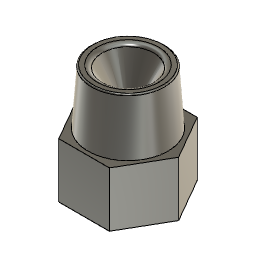
TubeNut175 (Autodesk Fusion 360 design; units mm, degrees)
Autodesk Fusion 360 part; units mm, degrees
note: some values were not read from the file. Set by a fixed rule: which sketch regions a step uses.
sketch "Sketch1" plane through (0, 0, 0) normal (0, 1, 0) x (1, 0, 0)
  circle A0 centre (0, 0) radius 8
  circle A1 centre (0, 0) radius 4
  circle A2 centre (0, 0) radius 1
  line L0 (4.6188, -8) -> (9.2376, 0)
  line L1 (9.2376, 0) -> (4.6188, 8)
  line L2 (4.6188, 8) -> (-4.6188, 8)
  line L3 (-4.6188, 8) -> (-9.2376, 0)
  line L4 (-9.2376, 0) -> (-4.6188, -8)
  line L5 (-4.6188, -8) -> (4.6188, -8)
  dimension "d1_1" = 16
  dimension "d4_1" = 8
  dimension "d7_1" = 2
  constraint coincident A0.centre A1.centre
  constraint concentric A0 A1
  measures "d1_1" diameter of A0
  measures "d4_1" diameter of A1
  measures "d7_1" diameter of A2
extrude "Extrude1" add sketch "Sketch1" along normal blind 20 draft -4 contours A0 | A1 | A2
extrude "Extrude4" add sketch "Sketch1" along normal blind 10 contours A0 | A0 L0 L1 | A0 L1 L2 | A0 L0 L5 | A0 L2 L3 | A0 L4 L5 | A0 L3 L4 | A1 | A2
extrude "Extrude3" cut sketch "Sketch1" along normal through all contours A2
chamfer "Chamfer1" distance 4 angle 60 1 edges at (-0.9323, 20, -0.3616) measured on face at (4.706, 20, -0.3776)
fillet "Fillet1" radius 1 1 edges at (-4.6616, 20, 1.8081)
fillet "Fillet2" radius 3 1 edges at (-0.9323, 13.0718, -0.3616)
fillet "Fillet3" radius 0.25 1 edges at (-6.1547, 20, -2.3872)
sketch "Sketch2" plane through (0, 0, 0) normal (0, 0, 1) x (1, 0, 0)
  line L0 (0, 24) -> (0, -24) construction
  line L1 (-21.801, 0) -> (21.801, 0) construction
  line L2 (-4.5, 0) -> (-4.5, 8)
  line L3 (-4.5, 8) -> (0, 12.5)
  line L4 (0, 12.5) -> (0, 0)
  line L5 (-4.5, 0) -> (0, 0)
  dimension "d16" = 45
  dimension "d17" = 4.5
  dimension "d23" = 8
  constraint horizontal L1
  constraint vertical L0
  constraint coincident L4.end L5.end
  constraint coincident L0 L3.end
  constraint midpoint L4.end L1
  constraint perpendicular L0 L5
  constraint midpoint L4.end L0
  measures "d16" angle of L0 L3
  measures "d17" distance of L0 L2
  measures "d23" distance of L2.start L2.end
revolve "Revolve1" cut sketch "Sketch2" angle 360 about axis through (0, 24, 0) along (0, -1, 0)
fillet "Fillet4" radius 1 1 edges at (-0.9323, 11.5, -0.3616)
move_body "Move1" bodies 1 to x (1, 0, 0) y (0, 1, 0) z (0, 0, 1) at (40, 0, 0)
move_body "Move2" bodies 1 to x (1, 0, 0) y (0, 0, 1) z (0, -1, 0) at (0, 5, -5)
equation "d17 = BSP / 2"
equation "BSP = 9 mm"
